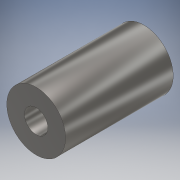
# Autodesk Inventor part: 778
Saved by Autodesk Inventor 2018.1 (Build 221171000, 171)
## iProperties
Created: 2023-04-05
Part Number: 778
Material: Сталь, углеродистая
Document SubType Name: ЛистМат
Designer: student
Density: 7.85 g/cm^3
Sheet Metal Rule: По умолчанию
Appearance: С умеренной полировкой
Author: student
Autodesk Inventor part; units mm, degrees
note: some values were not read from the file. Chosen so that the rebuilt part matches the saved one: edges of "Фаска1".
ref_plane "YZ Plane" through (0, 0, 0) normal (1, 0, 0) x (0, 1, 0)
ref_plane "XZ Plane" through (0, 0, 0) normal (0, 1, 0) x (-1, 0, 0)
ref_plane "XY Plane" through (0, 0, 0) normal (0, 0, 1) x (1, 0, 0)
sketch "Эскиз1" plane through (0, 0, 0) normal (0, 1, 0) x (-1, 0, 0)
  circle A0 centre (0, 0) radius 15
  dimension "d0" = 30
  constraints: 1 centre point, 1 coincident
  measures "d0" diameter of A0
extrude "Выдавливание1" add sketch "Эскиз1" along normal blind 55
hole "Отверстие1" at (0, 55, 0) direction (0, -1, 0) diameter 20 depth 25
hole "Отверстие2" at (0, 0, 0) direction (0, 1, 0) diameter 12 depth 30
thread "Резьба1" size "M20x2.5" class "6H" standard "ANSI Metric M Profile" length 20
chamfer "Фаска1" distance 2 angle 45 1 edges at (0, 30, -10)
chamfer "Фаска2" distance 1 angle 45 1 edges at (0, 55, -10)
equation "\"Радиус_гибки\" = Толщина"
equation "\"Ширина_просечки\" = Толщина"
equation "\"Глубина_просечки\" = 0.5 * Толщина"
equation "\"Размер_просечки\" = 4 * Толщина"
equation "\"Мин_остаток\" = 2 * Толщина"
equation "\"Радиус_перехода\" = Радиус_гибки"
equation "\"Радиус_Якоби\" = Толщина"
equation "\"Размер_зазора\" = Толщина"
equation "\"Толщина\" = 3.048"
